Autodesk Inventor part; units mm, degrees
(part 3 of 6)
  line L1057 (-22.5678, -22.0282) -> (-22.8077, -22.2961) construction
  spline S252 degree 2 poles (-22.8077, -22.2961) (-23.0757, -22.5921) (-23.5275, -22.5921) knots 0 0 0 1 1 1
  line L1058 (-22.8077, -22.2961) -> (-23.0757, -22.5921) construction
  line L1059 (-23.0757, -22.5921) -> (-23.5275, -22.5921) construction
  line L1060 (-23.5275, -22.5921) -> (-23.7675, -22.5921)
  spline S253 degree 2 poles (-23.7675, -22.5921) (-24.2553, -22.5921) (-24.6272, -22.3041) knots 0 0 0 1 1 1
  line L1061 (-23.7675, -22.5921) -> (-24.2553, -22.5921) construction
  line L1062 (-24.2553, -22.5921) -> (-24.6272, -22.3041) construction
  spline S254 degree 2 poles (-24.6272, -22.3041) (-24.7272, -22.2282) (-24.7272, -22.1162) knots 0 0 0 1 1 1
  line L1063 (-24.6272, -22.3041) -> (-24.7272, -22.2282) construction
  line L1064 (-24.7272, -22.2282) -> (-24.7272, -22.1162) construction
  spline S255 degree 2 poles (-24.7272, -22.1162) (-24.7272, -22.0162) (-24.5832, -21.8683) (-24.4873, -21.8683) knots 0 0 0 1 2 2 2
  line L1065 (-24.7272, -22.1162) -> (-24.7272, -22.0162) construction
  line L1066 (-24.7272, -22.0162) -> (-24.5832, -21.8683) construction
  line L1067 (-24.5832, -21.8683) -> (-24.4873, -21.8683) construction
  spline S256 degree 2 poles (-24.4873, -21.8683) (-24.4113, -21.8683) (-24.3393, -21.9202) knots 0 0 0 1 1 1
  line L1068 (-24.4873, -21.8683) -> (-24.4113, -21.8683) construction
  line L1069 (-24.4113, -21.8683) -> (-24.3393, -21.9202) construction
  spline S257 degree 2 poles (-24.3393, -21.9202) (-24.0914, -22.1122) (-23.7675, -22.1122) knots 0 0 0 1 1 1
  line L1070 (-24.3393, -21.9202) -> (-24.0914, -22.1122) construction
  line L1071 (-24.0914, -22.1122) -> (-23.7675, -22.1122) construction
  line L1072 (-23.7675, -22.1122) -> (-23.5275, -22.1122)
  spline S258 degree 2 poles (-23.5275, -22.1122) (-23.2996, -22.1122) (-23.1676, -21.9602) knots 0 0 0 1 1 1
  line L1073 (-23.5275, -22.1122) -> (-23.2996, -22.1122) construction
  line L1074 (-23.2996, -22.1122) -> (-23.1676, -21.9602) construction
  spline S259 degree 2 poles (-23.1676, -21.9602) (-23.0477, -21.8243) (-23.0477, -21.6283) knots 0 0 0 1 1 1
  line L1075 (-23.1676, -21.9602) -> (-23.0477, -21.8243) construction
  line L1076 (-23.0477, -21.8243) -> (-23.0477, -21.6283) construction
  spline S260 degree 2 poles (-23.0477, -21.6283) (-23.0477, -21.2005) (-23.4635, -21.1565) knots 0 0 0 1 1 1
  line L1077 (-23.0477, -21.6283) -> (-23.0477, -21.2005) construction
  line L1078 (-23.0477, -21.2005) -> (-23.4635, -21.1565) construction
  line L1079 (-23.4635, -21.1565) -> (-23.7635, -21.1565)
  spline S261 degree 2 poles (10.7013, -8.7285) (10.4614, -8.7285) (10.4614, -8.4886) knots 0 0 0 1 1 1
  line L1080 (10.7013, -8.7285) -> (10.4614, -8.7285) construction
  line L1081 (10.4614, -8.7285) -> (10.4614, -8.4886) construction
  line L1082 (10.4614, -8.4886) -> (10.4614, -6.3372)
  spline S262 degree 2 poles (10.4614, -6.3372) (10.4614, -6.1413) (10.1815, -5.8573) (9.9855, -5.8573) knots 0 0 0 1 2 2 2
  line L1083 (10.4614, -6.3372) -> (10.4614, -6.1413) construction
  line L1084 (10.4614, -6.1413) -> (10.1815, -5.8573) construction
  line L1085 (10.1815, -5.8573) -> (9.9855, -5.8573) construction
  spline S263 degree 2 poles (9.0298, -8.4886) (9.0298, -8.7285) (8.7899, -8.7285) knots 0 0 0 1 1 1
  line L1086 (9.0298, -8.4886) -> (9.0298, -8.7285) construction
  line L1087 (9.0298, -8.7285) -> (8.7899, -8.7285) construction
  spline S264 degree 2 poles (8.7899, -8.7285) (8.5499, -8.7285) (8.5499, -8.4886) knots 0 0 0 1 1 1
  line L1088 (8.7899, -8.7285) -> (8.5499, -8.7285) construction
  line L1089 (8.5499, -8.7285) -> (8.5499, -8.4886) construction
  line L1090 (8.5499, -8.4886) -> (8.5499, -5.6174)
  spline S265 degree 2 poles (8.5499, -5.6174) (8.5499, -5.3775) (8.7899, -5.3775) knots 0 0 0 1 1 1
  line L1091 (8.5499, -5.6174) -> (8.5499, -5.3775) construction
  line L1092 (8.5499, -5.3775) -> (8.7899, -5.3775) construction
  line L1093 (8.7899, -5.3775) -> (9.9855, -5.3775)
  spline S266 degree 2 poles (9.9855, -5.3775) (10.3814, -5.3775) (10.9413, -5.9373) (10.9413, -6.3332) knots 0 0 0 1 2 2 2
  line L1094 (9.9855, -5.3775) -> (10.3814, -5.3775) construction
  line L1095 (10.3814, -5.3775) -> (10.9413, -5.9373) construction
  line L1096 (10.9413, -5.9373) -> (10.9413, -6.3332) construction
  line L1097 (10.9413, -6.3332) -> (10.9413, -8.4886)
  spline S267 degree 2 poles (10.9413, -8.4886) (10.9413, -8.7285) (10.7013, -8.7285) knots 0 0 0 1 1 1
  line L1098 (10.9413, -8.4886) -> (10.9413, -8.7285) construction
  line L1099 (10.9413, -8.7285) -> (10.7013, -8.7285) construction
  spline S268 degree 2 poles (6.6345, -8.2487) (6.8304, -8.2487) (7.1103, -7.9647) (7.1103, -7.7688) knots 0 0 0 1 2 2 2
  line L1100 (6.6345, -8.2487) -> (6.8304, -8.2487) construction
  line L1101 (6.8304, -8.2487) -> (7.1103, -7.9647) construction
  line L1102 (7.1103, -7.9647) -> (7.1103, -7.7688) construction
  spline S269 degree 2 poles (6.1546, -5.8573) (5.9587, -5.8573) (5.6787, -6.1413) (5.6787, -6.3372) knots 0 0 0 1 2 2 2
  line L1103 (6.1546, -5.8573) -> (5.9587, -5.8573) construction
  line L1104 (5.9587, -5.8573) -> (5.6787, -6.1413) construction
  line L1105 (5.6787, -6.1413) -> (5.6787, -6.3372) construction
  line L1106 (5.6787, -6.3372) -> (5.6787, -7.7688)
  spline S270 degree 2 poles (5.6787, -7.7688) (5.6787, -7.9647) (5.9587, -8.2487) (6.1546, -8.2487) knots 0 0 0 1 2 2 2
  line L1107 (5.6787, -7.7688) -> (5.6787, -7.9647) construction
  line L1108 (5.6787, -7.9647) -> (5.9587, -8.2487) construction
  line L1109 (5.9587, -8.2487) -> (6.1546, -8.2487) construction
  line L1110 (6.1546, -8.2487) -> (6.6345, -8.2487)
  line L1111 (6.6345, -8.7285) -> (6.1546, -8.7285)
  spline S271 degree 2 poles (6.1546, -8.7285) (5.7627, -8.7285) (5.1989, -8.1687) (5.1989, -7.7728) knots 0 0 0 1 2 2 2
  line L1112 (6.1546, -8.7285) -> (5.7627, -8.7285) construction
  line L1113 (5.7627, -8.7285) -> (5.1989, -8.1687) construction
  line L1114 (5.1989, -8.1687) -> (5.1989, -7.7728) construction
  line L1115 (5.1989, -7.7728) -> (5.1989, -6.3332)
  spline S272 degree 2 poles (5.1989, -6.3332) (5.1989, -5.9373) (5.7627, -5.3775) (6.1546, -5.3775) knots 0 0 0 1 2 2 2
  line L1116 (5.1989, -6.3332) -> (5.1989, -5.9373) construction
  line L1117 (5.1989, -5.9373) -> (5.7627, -5.3775) construction
  line L1118 (5.7627, -5.3775) -> (6.1546, -5.3775) construction
  line L1119 (6.1546, -5.3775) -> (7.3503, -5.3775)
  spline S273 degree 2 poles (7.3503, -5.3775) (7.5902, -5.3775) (7.5902, -5.6174) knots 0 0 0 1 1 1
  line L1120 (7.3503, -5.3775) -> (7.5902, -5.3775) construction
  line L1121 (7.5902, -5.3775) -> (7.5902, -5.6174) construction
  line L1122 (7.5902, -5.6174) -> (7.5902, -7.7648)
  spline S274 degree 2 poles (7.5902, -7.7648) (7.5902, -8.1247) (7.9261, -8.2687) knots 0 0 0 1 1 1
  line L1123 (7.5902, -7.7648) -> (7.5902, -8.1247) construction
  line L1124 (7.5902, -8.1247) -> (7.9261, -8.2687) construction
  spline S275 degree 2 poles (7.9261, -8.2687) (8.0741, -8.3286) (8.0741, -8.4806) knots 0 0 0 1 1 1
  line L1125 (7.9261, -8.2687) -> (8.0741, -8.3286) construction
  line L1126 (8.0741, -8.3286) -> (8.0741, -8.4806) construction
  spline S276 degree 2 poles (8.0741, -8.4806) (8.0741, -8.5806) (7.9381, -8.7325) (7.8381, -8.7325) knots 0 0 0 1 2 2 2
  line L1127 (8.0741, -8.4806) -> (8.0741, -8.5806) construction
  line L1128 (8.0741, -8.5806) -> (7.9381, -8.7325) construction
  line L1129 (7.9381, -8.7325) -> (7.8381, -8.7325) construction
  spline S277 degree 2 poles (7.8381, -8.7325) (7.7861, -8.7325) (7.7342, -8.7085) knots 0 0 0 1 1 1
  line L1130 (7.8381, -8.7325) -> (7.7861, -8.7325) construction
  line L1131 (7.7861, -8.7325) -> (7.7342, -8.7085) construction
  spline S278 degree 2 poles (7.7342, -8.7085) (7.4942, -8.6046) (7.3463, -8.4126) knots 0 0 0 1 1 1
  line L1132 (7.7342, -8.7085) -> (7.4942, -8.6046) construction
  line L1133 (7.4942, -8.6046) -> (7.3463, -8.4126) construction
  spline S279 degree 2 poles (7.3463, -8.4126) (7.0583, -8.7285) (6.6345, -8.7285) knots 0 0 0 1 1 1
  line L1134 (7.3463, -8.4126) -> (7.0583, -8.7285) construction
  line L1135 (7.0583, -8.7285) -> (6.6345, -8.7285) construction
  spline S280 degree 2 poles (8.5987, 1.0626) (8.3588, 1.0626) (8.3588, 1.3026) knots 0 0 0 1 1 1
  line L1136 (8.5987, 1.0626) -> (8.3588, 1.0626) construction
  line L1137 (8.3588, 1.0626) -> (8.3588, 1.3026) construction
  line L1138 (8.3588, 1.3026) -> (8.3588, 3.454)
  spline S281 degree 2 poles (8.3588, 3.454) (8.3588, 3.6499) (8.0788, 3.9338) (7.8829, 3.9338) knots 0 0 0 1 2 2 2
  line L1139 (8.3588, 3.454) -> (8.3588, 3.6499) construction
  line L1140 (8.3588, 3.6499) -> (8.0788, 3.9338) construction
  line L1141 (8.0788, 3.9338) -> (7.8829, 3.9338) construction
  spline S282 degree 2 poles (6.9272, 1.3026) (6.9272, 1.0626) (6.6872, 1.0626) knots 0 0 0 1 1 1
  line L1142 (6.9272, 1.3026) -> (6.9272, 1.0626) construction
  line L1143 (6.9272, 1.0626) -> (6.6872, 1.0626) construction
  spline S283 degree 2 poles (6.6872, 1.0626) (6.4473, 1.0626) (6.4473, 1.3026) knots 0 0 0 1 1 1
  line L1144 (6.6872, 1.0626) -> (6.4473, 1.0626) construction
  line L1145 (6.4473, 1.0626) -> (6.4473, 1.3026) construction
  line L1146 (6.4473, 1.3026) -> (6.4473, 4.1738)
  spline S284 degree 2 poles (6.4473, 4.1738) (6.4473, 4.4137) (6.6872, 4.4137) knots 0 0 0 1 1 1
  line L1147 (6.4473, 4.1738) -> (6.4473, 4.4137) construction
  line L1148 (6.4473, 4.4137) -> (6.6872, 4.4137) construction
  line L1149 (6.6872, 4.4137) -> (7.8829, 4.4137)
  spline S285 degree 2 poles (7.8829, 4.4137) (8.2788, 4.4137) (8.8386, 3.8539) (8.8386, 3.458) knots 0 0 0 1 2 2 2
  line L1150 (7.8829, 4.4137) -> (8.2788, 4.4137) construction
  line L1151 (8.2788, 4.4137) -> (8.8386, 3.8539) construction
  line L1152 (8.8386, 3.8539) -> (8.8386, 3.458) construction
  line L1153 (8.8386, 3.458) -> (8.8386, 1.3026)
  spline S286 degree 2 poles (8.8386, 1.3026) (8.8386, 1.0626) (8.5987, 1.0626) knots 0 0 0 1 1 1
  line L1154 (8.8386, 1.3026) -> (8.8386, 1.0626) construction
  line L1155 (8.8386, 1.0626) -> (8.5987, 1.0626) construction
  spline S287 degree 2 poles (-14.2805, -7.629) (-14.6764, -7.629) (-15.2362, -7.0692) (-15.2362, -6.6733) knots 0 0 0 1 2 2 2
  line L1156 (-14.2805, -7.629) -> (-14.6764, -7.629) construction
  line L1157 (-14.6764, -7.629) -> (-15.2362, -7.0692) construction
  line L1158 (-15.2362, -7.0692) -> (-15.2362, -6.6733) construction
  line L1159 (-15.2362, -6.6733) -> (-15.2362, -4.9978)
  spline S288 degree 2 poles (-15.2362, -4.9978) (-15.2362, -4.7578) (-14.9963, -4.7578) knots 0 0 0 1 1 1
  line L1160 (-15.2362, -4.9978) -> (-15.2362, -4.7578) construction
  line L1161 (-15.2362, -4.7578) -> (-14.9963, -4.7578) construction
  spline S289 degree 2 poles (-14.9963, -4.7578) (-14.7563, -4.7578) (-14.7563, -4.9978) knots 0 0 0 1 1 1
  line L1162 (-14.9963, -4.7578) -> (-14.7563, -4.7578) construction
  line L1163 (-14.7563, -4.7578) -> (-14.7563, -4.9978) construction
  line L1164 (-14.7563, -4.9978) -> (-14.7563, -6.6693)
  spline S290 degree 2 poles (-14.7563, -6.6693) (-14.7563, -6.8652) (-14.4724, -7.1491) (-14.2765, -7.1491) knots 0 0 0 1 2 2 2
  line L1165 (-14.7563, -6.6693) -> (-14.7563, -6.8652) construction
  line L1166 (-14.7563, -6.8652) -> (-14.4724, -7.1491) construction
  line L1167 (-14.4724, -7.1491) -> (-14.2765, -7.1491) construction
  spline S291 degree 2 poles (-12.8449, -4.9978) (-12.8449, -4.7578) (-12.6049, -4.7578) knots 0 0 0 1 1 1
  line L1168 (-12.8449, -4.9978) -> (-12.8449, -4.7578) construction
  line L1169 (-12.8449, -4.7578) -> (-12.6049, -4.7578) construction
  spline S292 degree 2 poles (-12.6049, -4.7578) (-12.365, -4.7578) (-12.365, -4.9978) knots 0 0 0 1 1 1
  line L1170 (-12.6049, -4.7578) -> (-12.365, -4.7578) construction
  line L1171 (-12.365, -4.7578) -> (-12.365, -4.9978) construction
  line L1172 (-12.365, -4.9978) -> (-12.365, -8.5887)
  spline S293 degree 2 poles (-12.365, -8.5887) (-12.365, -8.9846) (-12.9249, -9.5445) (-13.3207, -9.5445) knots 0 0 0 1 2 2 2
  line L1173 (-12.365, -8.5887) -> (-12.365, -8.9846) construction
  line L1174 (-12.365, -8.9846) -> (-12.9249, -9.5445) construction
  line L1175 (-12.9249, -9.5445) -> (-13.3207, -9.5445) construction
  line L1176 (-13.3207, -9.5445) -> (-14.5164, -9.5445)
  spline S294 degree 2 poles (-14.5164, -9.5445) (-14.7563, -9.5445) (-14.7563, -9.3045) knots 0 0 0 1 1 1
  line L1177 (-14.5164, -9.5445) -> (-14.7563, -9.5445) construction
  line L1178 (-14.7563, -9.5445) -> (-14.7563, -9.3045) construction
  spline S295 degree 2 poles (-14.7563, -9.3045) (-14.7563, -9.0646) (-14.5164, -9.0646) knots 0 0 0 1 1 1
  line L1179 (-14.7563, -9.3045) -> (-14.7563, -9.0646) construction
  line L1180 (-14.7563, -9.0646) -> (-14.5164, -9.0646) construction
  line L1181 (-14.5164, -9.0646) -> (-13.3207, -9.0646)
  spline S296 degree 2 poles (-13.3207, -9.0646) (-13.1248, -9.0646) (-12.8449, -8.7807) (-12.8449, -8.5847) knots 0 0 0 1 2 2 2
  line L1182 (-13.3207, -9.0646) -> (-13.1248, -9.0646) construction
  line L1183 (-13.1248, -9.0646) -> (-12.8449, -8.7807) construction
  line L1184 (-12.8449, -8.7807) -> (-12.8449, -8.5847) construction
  spline S297 degree 2 poles (-20.2548, -6.6733) (-20.0189, -6.6733) (-20.0189, -6.9132) knots 0 0 0 1 1 1
  line L1185 (-20.2548, -6.6733) -> (-20.0189, -6.6733) construction
  line L1186 (-20.0189, -6.6733) -> (-20.0189, -6.9132) construction
  spline S298 degree 2 poles (-20.0189, -6.9132) (-20.0189, -7.1531) (-20.2548, -7.1531) knots 0 0 0 1 1 1
  line L1187 (-20.0189, -6.9132) -> (-20.0189, -7.1531) construction
  line L1188 (-20.0189, -7.1531) -> (-20.2548, -7.1531) construction
  spline S299 degree 2 poles (-19.7789, -9.0646) (-19.539, -9.0646) (-19.539, -9.3045) knots 0 0 0 1 1 1
  line L1189 (-19.7789, -9.0646) -> (-19.539, -9.0646) construction
  line L1190 (-19.539, -9.0646) -> (-19.539, -9.3045) construction
  spline S300 degree 2 poles (-19.539, -9.3045) (-19.539, -9.5445) (-19.7789, -9.5445) knots 0 0 0 1 1 1
  line L1191 (-19.539, -9.3045) -> (-19.539, -9.5445) construction
  line L1192 (-19.539, -9.5445) -> (-19.7789, -9.5445) construction
  line L1193 (-19.7789, -9.5445) -> (-21.6984, -9.5445)
  spline S301 degree 2 poles (-21.6984, -9.5445) (-21.9383, -9.5445) (-21.9383, -9.3205) knots 0 0 0 1 1 1
  line L1194 (-21.6984, -9.5445) -> (-21.9383, -9.5445) construction
  line L1195 (-21.9383, -9.5445) -> (-21.9383, -9.3205) construction
  line L1196 (-21.9383, -9.3205) -> (-21.9383, -4.9978)
  spline S302 degree 2 poles (-21.9383, -4.9978) (-21.9383, -4.7578) (-21.6984, -4.7578) knots 0 0 0 1 1 1
  line L1197 (-21.9383, -4.9978) -> (-21.9383, -4.7578) construction
  line L1198 (-21.9383, -4.7578) -> (-21.6984, -4.7578) construction
  line L1199 (-21.6984, -4.7578) -> (-19.7789, -4.7578)
  spline S303 degree 2 poles (-19.7789, -4.7578) (-19.539, -4.7578) (-19.539, -4.9978) knots 0 0 0 1 1 1
  line L1200 (-19.7789, -4.7578) -> (-19.539, -4.7578) construction
  line L1201 (-19.539, -4.7578) -> (-19.539, -4.9978) construction
  spline S304 degree 2 poles (-19.539, -4.9978) (-19.539, -5.2377) (-19.7789, -5.2377) knots 0 0 0 1 1 1
  line L1202 (-19.539, -4.9978) -> (-19.539, -5.2377) construction
  line L1203 (-19.539, -5.2377) -> (-19.7789, -5.2377) construction
  spline S305 degree 2 poles (-19.9181, 7.2042) (-20.418, 7.2042) (-21.1178, 7.904) (-21.1178, 8.3999) knots 0 0 0 1 2 2 2
  line L1204 (-19.9181, 7.2042) -> (-20.418, 7.2042) construction
  line L1205 (-20.418, 7.2042) -> (-21.1178, 7.904) construction
  line L1206 (-21.1178, 7.904) -> (-21.1178, 8.3999) construction
  line L1207 (-21.1178, 8.3999) -> (-21.1178, 10.7952)
  spline S306 degree 2 poles (-21.1178, 10.7952) (-21.1178, 11.287) (-20.418, 11.9909) (-19.9181, 11.9909) knots 0 0 0 1 2 2 2
  line L1208 (-21.1178, 10.7952) -> (-21.1178, 11.287) construction
  line L1209 (-21.1178, 11.287) -> (-20.418, 11.9909) construction
  line L1210 (-20.418, 11.9909) -> (-19.9181, 11.9909) construction
  line L1211 (-19.9181, 11.9909) -> (-18.9624, 11.9909)
  spline S307 degree 2 poles (-18.9624, 11.9909) (-18.7225, 11.9909) (-18.7225, 11.7509) knots 0 0 0 1 1 1
  line L1212 (-18.9624, 11.9909) -> (-18.7225, 11.9909) construction
  line L1213 (-18.7225, 11.9909) -> (-18.7225, 11.7509) construction
  spline S308 degree 2 poles (-18.7225, 11.7509) (-18.7225, 11.511) (-18.9624, 11.511) knots 0 0 0 1 1 1
  line L1214 (-18.7225, 11.7509) -> (-18.7225, 11.511) construction
  line L1215 (-18.7225, 11.511) -> (-18.9624, 11.511) construction
  line L1216 (-18.9624, 11.511) -> (-19.9181, 11.511)
  spline S309 degree 2 poles (-19.9181, 11.511) (-20.218, 11.511) (-20.6379, 11.0911) (-20.6379, 10.7952) knots 0 0 0 1 2 2 2
  line L1217 (-19.9181, 11.511) -> (-20.218, 11.511) construction
  line L1218 (-20.218, 11.511) -> (-20.6379, 11.0911) construction
  line L1219 (-20.6379, 11.0911) -> (-20.6379, 10.7952) construction
  line L1220 (-20.6379, 10.7952) -> (-20.6379, 8.3999)
  spline S310 degree 2 poles (-20.6379, 8.3999) (-20.6379, 8.1039) (-20.218, 7.6841) (-19.9181, 7.6841) knots 0 0 0 1 2 2 2
  line L1221 (-20.6379, 8.3999) -> (-20.6379, 8.1039) construction
  line L1222 (-20.6379, 8.1039) -> (-20.218, 7.6841) construction
  line L1223 (-20.218, 7.6841) -> (-19.9181, 7.6841) construction
  line L1224 (-19.9181, 7.6841) -> (-18.9624, 7.6841)
  spline S311 degree 2 poles (-18.9624, 7.6841) (-18.7225, 7.6841) (-18.7225, 7.4441) knots 0 0 0 1 1 1
  line L1225 (-18.9624, 7.6841) -> (-18.7225, 7.6841) construction
  line L1226 (-18.7225, 7.6841) -> (-18.7225, 7.4441) construction
  spline S312 degree 2 poles (-18.7225, 7.4441) (-18.7225, 7.2042) (-18.9624, 7.2042) knots 0 0 0 1 1 1
  line L1227 (-18.7225, 7.4441) -> (-18.7225, 7.2042) construction
  line L1228 (-18.7225, 7.2042) -> (-18.9624, 7.2042) construction
  line L1229 (-18.9624, 7.2042) -> (-19.9181, 7.2042)
  spline S313 degree 2 poles (-10.2251, 1.4084) (-10.0292, 1.4084) (-9.7493, 1.6923) (-9.7493, 1.8882) knots 0 0 0 1 2 2 2
  line L1230 (-10.2251, 1.4084) -> (-10.0292, 1.4084) construction
  line L1231 (-10.0292, 1.4084) -> (-9.7493, 1.6923) construction
  line L1232 (-9.7493, 1.6923) -> (-9.7493, 1.8882) construction
  line L1233 (-9.7493, 1.8882) -> (-9.7493, 3.3198)
  spline S314 degree 2 poles (-9.7493, 3.3198) (-9.7493, 3.5158) (-10.0292, 3.7997) (-10.2251, 3.7997) knots 0 0 0 1 2 2 2
  line L1234 (-9.7493, 3.3198) -> (-9.7493, 3.5158) construction
  line L1235 (-9.7493, 3.5158) -> (-10.0292, 3.7997) construction
  line L1236 (-10.0292, 3.7997) -> (-10.2251, 3.7997) construction
  spline S315 degree 2 poles (-11.1809, -0.2671) (-11.1809, -0.5071) (-11.4208, -0.5071) knots 0 0 0 1 1 1
  line L1237 (-11.1809, -0.2671) -> (-11.1809, -0.5071) construction
  line L1238 (-11.1809, -0.5071) -> (-11.4208, -0.5071) construction
  spline S316 degree 2 poles (-11.4208, -0.5071) (-11.6607, -0.5071) (-11.6607, -0.2671) knots 0 0 0 1 1 1
  line L1239 (-11.4208, -0.5071) -> (-11.6607, -0.5071) construction
  line L1240 (-11.6607, -0.5071) -> (-11.6607, -0.2671) construction
  line L1241 (-11.6607, -0.2671) -> (-11.6607, 4.0396)
  spline S317 degree 2 poles (-11.6607, 4.0396) (-11.6607, 4.2796) (-11.4208, 4.2796) knots 0 0 0 1 1 1
  line L1242 (-11.6607, 4.0396) -> (-11.6607, 4.2796) construction
  line L1243 (-11.6607, 4.2796) -> (-11.4208, 4.2796) construction
  line L1244 (-11.4208, 4.2796) -> (-10.2251, 4.2796)
  spline S318 degree 2 poles (-10.2251, 4.2796) (-9.8293, 4.2796) (-9.2694, 3.7197) (-9.2694, 3.3238) knots 0 0 0 1 2 2 2
  line L1245 (-10.2251, 4.2796) -> (-9.8293, 4.2796) construction
  line L1246 (-9.8293, 4.2796) -> (-9.2694, 3.7197) construction
  line L1247 (-9.2694, 3.7197) -> (-9.2694, 3.3238) construction
  line L1248 (-9.2694, 3.3238) -> (-9.2694, 1.8842)
  spline S319 degree 2 poles (-9.2694, 1.8842) (-9.2694, 1.4884) (-9.8293, 0.9285) (-10.2251, 0.9285) knots 0 0 0 1 2 2 2
  line L1249 (-9.2694, 1.8842) -> (-9.2694, 1.4884) construction
  line L1250 (-9.2694, 1.4884) -> (-9.8293, 0.9285) construction
  line L1251 (-9.8293, 0.9285) -> (-10.2251, 0.9285) construction
  spline S320 degree 2 poles (-19.8024, 4.0396) (-19.8024, 4.2796) (-19.5625, 4.2796) knots 0 0 0 1 1 1
  line L1252 (-19.8024, 4.0396) -> (-19.8024, 4.2796) construction
  line L1253 (-19.8024, 4.2796) -> (-19.5625, 4.2796) construction
  spline S321 degree 2 poles (-19.5625, 4.2796) (-19.3226, 4.2796) (-19.3226, 4.0396) knots 0 0 0 1 1 1
  line L1254 (-19.5625, 4.2796) -> (-19.3226, 4.2796) construction
  line L1255 (-19.3226, 4.2796) -> (-19.3226, 4.0396) construction
  line L1256 (-19.3226, 4.0396) -> (-19.3226, 1.1685)
  spline S322 degree 2 poles (-19.3226, 1.1685) (-19.3226, 0.9285) (-19.5625, 0.9285) knots 0 0 0 1 1 1
  line L1257 (-19.3226, 1.1685) -> (-19.3226, 0.9285) construction
  line L1258 (-19.3226, 0.9285) -> (-19.5625, 0.9285) construction
  spline S323 degree 2 poles (-19.5625, 0.9285) (-19.8024, 0.9285) (-19.8024, 1.1685) knots 0 0 0 1 1 1
  line L1259 (-19.5625, 0.9285) -> (-19.8024, 0.9285) construction
  line L1260 (-19.8024, 0.9285) -> (-19.8024, 1.1685) construction
  spline S324 degree 2 poles (-21.234, 1.1685) (-21.234, 0.9285) (-21.474, 0.9285) knots 0 0 0 1 1 1
  line L1261 (-21.234, 1.1685) -> (-21.234, 0.9285) construction
  line L1262 (-21.234, 0.9285) -> (-21.474, 0.9285) construction
  spline S325 degree 2 poles (-21.474, 0.9285) (-21.7139, 0.9285) (-21.7139, 1.1685) knots 0 0 0 1 1 1
  line L1263 (-21.474, 0.9285) -> (-21.7139, 0.9285) construction
  line L1264 (-21.7139, 0.9285) -> (-21.7139, 1.1685) construction
  line L1265 (-21.7139, 1.1685) -> (-21.7139, 4.0396)
  spline S326 degree 2 poles (-21.7139, 4.0396) (-21.7139, 4.2796) (-21.474, 4.2796) knots 0 0 0 1 1 1
  line L1266 (-21.7139, 4.0396) -> (-21.7139, 4.2796) construction
  line L1267 (-21.7139, 4.2796) -> (-21.474, 4.2796) construction
  spline S327 degree 2 poles (-21.474, 4.2796) (-21.234, 4.2796) (-21.234, 4.0396) knots 0 0 0 1 1 1
  line L1268 (-21.474, 4.2796) -> (-21.234, 4.2796) construction
  line L1269 (-21.234, 4.2796) -> (-21.234, 4.0396) construction
  line L1270 (-18.0648, 28.7283) -> (-16.6292, 28.7283)
  spline S328 degree 2 poles (-16.6292, 28.7283) (-16.3893, 28.7283) (-16.3893, 28.4883) knots 0 0 0 1 1 1
  line L1271 (-16.6292, 28.7283) -> (-16.3893, 28.7283) construction
  line L1272 (-16.3893, 28.7283) -> (-16.3893, 28.4883) construction
  spline S329 degree 2 poles (-22.3312, 37.5726) (-22.4482, 37.5726) (-22.6239, 37.7483) (-22.6239, 37.8654) knots 0 0 0 1 2 2 2
  line L1273 (-22.3312, 37.5726) -> (-22.4482, 37.5726) construction
  line L1274 (-22.4482, 37.5726) -> (-22.6239, 37.7483) construction
  line L1275 (-22.6239, 37.7483) -> (-22.6239, 37.8654) construction
  line L1276 (-22.6239, 37.8654) -> (-22.6239, 43.1196)
  spline S330 degree 2 poles (-22.6239, 43.1196) (-22.6239, 43.2367) (-22.4482, 43.4124) (-22.3312, 43.4124) knots 0 0 0 1 2 2 2
  line L1277 (-22.6239, 43.1196) -> (-22.6239, 43.2367) construction
  line L1278 (-22.6239, 43.2367) -> (-22.4482, 43.4124) construction
  line L1279 (-22.4482, 43.4124) -> (-22.3312, 43.4124) construction
  spline S331 degree 2 poles (14.945, 104.9441) (14.9341, 104.5681) (14.9069, 103.8762) (14.8906, 103.5983) knots 0 0 0 1 2 2 2
  line L1280 (14.945, 104.9441) -> (14.9341, 104.5681) construction
  line L1281 (14.9341, 104.5681) -> (14.9069, 103.8762) construction
  line L1282 (14.9069, 103.8762) -> (14.8906, 103.5983) construction
  spline S332 degree 2 poles (14.8906, 103.5983) (14.8633, 102.8899) (14.7325, 101.931) (14.6345, 101.6422) knots 0 0 0 1 2 2 2
  line L1283 (14.8906, 103.5983) -> (14.8633, 102.8899) construction
  line L1284 (14.8633, 102.8899) -> (14.7325, 101.931) construction
  line L1285 (14.7325, 101.931) -> (14.6345, 101.6422) construction
  spline S333 degree 2 poles (14.6345, 101.6422) (14.5364, 101.3425) (14.2966, 101.0101) (14.1441, 100.8739) knots 0 0 0 1 2 2 2
  line L1286 (14.6345, 101.6422) -> (14.5364, 101.3425) construction
  line L1287 (14.5364, 101.3425) -> (14.2966, 101.0101) construction
  line L1288 (14.2966, 101.0101) -> (14.1441, 100.8739) construction
  spline S334 degree 2 poles (14.1441, 100.8739) (13.9915, 100.7377) (13.6428, 100.6015) (13.4194, 100.6015) knots 0 0 0 1 2 2 2
  line L1289 (14.1441, 100.8739) -> (13.9915, 100.7377) construction
  line L1290 (13.9915, 100.7377) -> (13.6428, 100.6015) construction
  line L1291 (13.6428, 100.6015) -> (13.4194, 100.6015) construction
  spline S335 degree 2 poles (13.4194, 100.6015) (13.3486, 100.6015) (13.1197, 100.6124) (13.0761, 100.6124) knots 0 0 0 1 2 2 2
  line L1292 (13.4194, 100.6015) -> (13.3486, 100.6015) construction
  line L1293 (13.3486, 100.6015) -> (13.1197, 100.6124) construction
  line L1294 (13.1197, 100.6124) -> (13.0761, 100.6124) construction
  spline S336 degree 2 poles (13.1197, 101.3534) (13.1524, 101.3534) (13.2233, 101.3425) (13.2668, 101.3425) knots 0 0 0 1 2 2 2
  line L1295 (13.1197, 101.3534) -> (13.1524, 101.3534) construction
  line L1296 (13.1524, 101.3534) -> (13.2233, 101.3425) construction
  line L1297 (13.2233, 101.3425) -> (13.2668, 101.3425) construction
  spline S337 degree 2 poles (13.2668, 101.3425) (13.3758, 101.3425) (13.5829, 101.4079) (13.6646, 101.4896) knots 0 0 0 1 2 2 2
  line L1298 (13.2668, 101.3425) -> (13.3758, 101.3425) construction
  line L1299 (13.3758, 101.3425) -> (13.5829, 101.4079) construction
  line L1300 (13.5829, 101.4079) -> (13.6646, 101.4896) construction
  spline S338 degree 2 poles (13.6646, 101.4896) (13.888, 101.713) (14.095, 102.8191) (14.1386, 103.8162) knots 0 0 0 1 2 2 2
  line L1301 (13.6646, 101.4896) -> (13.888, 101.713) construction
  line L1302 (13.888, 101.713) -> (14.095, 102.8191) construction
  line L1303 (14.095, 102.8191) -> (14.1386, 103.8162) construction
  spline S339 degree 2 poles (14.1386, 103.8162) (14.1604, 104.1867) (14.1931, 105.1947) (14.204, 105.6579) knots 0 0 0 1 2 2 2
  line L1304 (14.1386, 103.8162) -> (14.1604, 104.1867) construction
  line L1305 (14.1604, 104.1867) -> (14.1931, 105.1947) construction
  line L1306 (14.1931, 105.1947) -> (14.204, 105.6579) construction
  spline S340 degree 2 poles (10.5043, 101.2008) (11.1582, 101.2008) (11.8774, 102.1653) (11.8774, 103.1351) knots 0 0 0 1 2 2 2
  line L1307 (10.5043, 101.2008) -> (11.1582, 101.2008) construction
  line L1308 (11.1582, 101.2008) -> (11.8774, 102.1653) construction
  line L1309 (11.8774, 102.1653) -> (11.8774, 103.1351) construction
  spline S341 degree 2 poles (11.8774, 103.1351) (11.8774, 104.1159) (11.1636, 105.0694) (10.5043, 105.0694) knots 0 0 0 1 2 2 2
  line L1310 (11.8774, 103.1351) -> (11.8774, 104.1159) construction
  line L1311 (11.8774, 104.1159) -> (11.1636, 105.0694) construction
  line L1312 (11.1636, 105.0694) -> (10.5043, 105.0694) construction
  spline S342 degree 2 poles (10.5043, 105.0694) (9.8451, 105.0694) (9.1258, 104.1159) (9.1258, 103.1351) knots 0 0 0 1 2 2 2
  line L1313 (10.5043, 105.0694) -> (9.8451, 105.0694) construction
  line L1314 (9.8451, 105.0694) -> (9.1258, 104.1159) construction
  line L1315 (9.1258, 104.1159) -> (9.1258, 103.1351) construction
  spline S343 degree 2 poles (9.1258, 103.1351) (9.1258, 102.1816) (9.8451, 101.2008) (10.5043, 101.2008) knots 0 0 0 1 2 2 2
  line L1316 (9.1258, 103.1351) -> (9.1258, 102.1816) construction
  line L1317 (9.1258, 102.1816) -> (9.8451, 101.2008) construction
  line L1318 (9.8451, 101.2008) -> (10.5043, 101.2008) construction
  spline S344 degree 2 poles (10.5043, 100.4707) (9.4527, 100.4707) (8.2486, 101.9037) (8.2486, 103.1351) knots 0 0 0 1 2 2 2
  line L1319 (10.5043, 100.4707) -> (9.4527, 100.4707) construction
  line L1320 (9.4527, 100.4707) -> (8.2486, 101.9037) construction
  line L1321 (8.2486, 101.9037) -> (8.2486, 103.1351) construction
  spline S345 degree 2 poles (8.2486, 103.1351) (8.2486, 104.3992) (9.4909, 105.7995) (10.5043, 105.7995) knots 0 0 0 1 2 2 2
  line L1322 (8.2486, 103.1351) -> (8.2486, 104.3992) construction
  line L1323 (8.2486, 104.3992) -> (9.4909, 105.7995) construction
  line L1324 (9.4909, 105.7995) -> (10.5043, 105.7995) construction
  spline S346 degree 2 poles (10.5043, 105.7995) (11.5287, 105.7995) (12.7547, 104.4047) (12.7547, 103.1351) knots 0 0 0 1 2 2 2
  line L1325 (10.5043, 105.7995) -> (11.5287, 105.7995) construction
  line L1326 (11.5287, 105.7995) -> (12.7547, 104.4047) construction
  line L1327 (12.7547, 104.4047) -> (12.7547, 103.1351) construction
  spline S347 degree 2 poles (12.7547, 103.1351) (12.7547, 101.8601) (11.5287, 100.4707) (10.5043, 100.4707) knots 0 0 0 1 2 2 2
  line L1328 (12.7547, 103.1351) -> (12.7547, 101.8601) construction
  line L1329 (12.7547, 101.8601) -> (11.5287, 100.4707) construction
  line L1330 (11.5287, 100.4707) -> (10.5043, 100.4707) construction
  spline S348 degree 2 poles (5.4588, 101.2771) (6.1181, 101.2771) (6.8483, 102.247) (6.8483, 103.1733) knots 0 0 0 1 2 2 2
  line L1331 (5.4588, 101.2771) -> (6.1181, 101.2771) construction
  line L1332 (6.1181, 101.2771) -> (6.8483, 102.247) construction
  line L1333 (6.8483, 102.247) -> (6.8483, 103.1733) construction
  spline S349 degree 2 poles (6.8483, 103.1733) (6.8483, 104.0396) (6.2979, 104.9931) (5.6822, 104.9931) knots 0 0 0 1 2 2 2
  line L1334 (6.8483, 103.1733) -> (6.8483, 104.0396) construction
  line L1335 (6.8483, 104.0396) -> (6.2979, 104.9931) construction
  line L1336 (6.2979, 104.9931) -> (5.6822, 104.9931) construction
  spline S350 degree 2 poles (5.6822, 104.9931) (5.3226, 104.9931) (4.647, 104.6717) (4.3473, 104.421) knots 0 0 0 1 2 2 2
  line L1337 (5.6822, 104.9931) -> (5.3226, 104.9931) construction
  line L1338 (5.3226, 104.9931) -> (4.647, 104.6717) construction
  line L1339 (4.647, 104.6717) -> (4.3473, 104.421) construction
  line L1340 (4.3473, 104.421) -> (4.3473, 101.555)
  spline S351 degree 2 poles (4.3473, 101.555) (4.6797, 101.397) (5.1537, 101.2771) (5.4588, 101.2771) knots 0 0 0 1 2 2 2
  line L1341 (4.3473, 101.555) -> (4.6797, 101.397) construction
  line L1342 (4.6797, 101.397) -> (5.1537, 101.2771) construction
  line L1343 (5.1537, 101.2771) -> (5.4588, 101.2771) construction
  spline S352 degree 2 poles (5.6005, 100.5143) (5.2246, 100.5143) (4.647, 100.6887) (4.3473, 100.8685) knots 0 0 0 1 2 2 2
  line L1344 (5.6005, 100.5143) -> (5.2246, 100.5143) construction
  line L1345 (5.2246, 100.5143) -> (4.647, 100.6887) construction
  line L1346 (4.647, 100.6887) -> (4.3473, 100.8685) construction
  spline S353 degree 2 poles (4.3473, 105.1294) (4.6633, 105.4181) (5.4371, 105.7995) (5.8893, 105.7995) knots 0 0 0 1 2 2 2
  line L1347 (4.3473, 105.1294) -> (4.6633, 105.4181) construction
  line L1348 (4.6633, 105.4181) -> (5.4371, 105.7995) construction
  line L1349 (5.4371, 105.7995) -> (5.8893, 105.7995) construction
  spline S354 degree 2 poles (5.8893, 105.7995) (6.7556, 105.7995) (7.7255, 104.4265) (7.7255, 103.2713) knots 0 0 0 1 2 2 2
  line L1350 (5.8893, 105.7995) -> (6.7556, 105.7995) construction
  line L1351 (6.7556, 105.7995) -> (7.7255, 104.4265) construction
  line L1352 (7.7255, 104.4265) -> (7.7255, 103.2713) construction
  spline S355 degree 2 poles (7.7255, 103.2713) (7.7255, 102.0072) (6.5213, 100.5143) (5.6005, 100.5143) knots 0 0 0 1 2 2 2
  line L1353 (7.7255, 103.2713) -> (7.7255, 102.0072) construction
  line L1354 (7.7255, 102.0072) -> (6.5213, 100.5143) construction
  line L1355 (6.5213, 100.5143) -> (5.6005, 100.5143) construction
  spline S356 degree 2 poles (-9.1437, 101.2008) (-8.4898, 101.2008) (-7.7706, 102.1653) (-7.7706, 103.1351) knots 0 0 0 1 2 2 2
  line L1356 (-9.1437, 101.2008) -> (-8.4898, 101.2008) construction
  line L1357 (-8.4898, 101.2008) -> (-7.7706, 102.1653) construction
  line L1358 (-7.7706, 102.1653) -> (-7.7706, 103.1351) construction
  spline S357 degree 2 poles (-7.7706, 103.1351) (-7.7706, 104.1159) (-8.4844, 105.0694) (-9.1437, 105.0694) knots 0 0 0 1 2 2 2
  line L1359 (-7.7706, 103.1351) -> (-7.7706, 104.1159) construction
  line L1360 (-7.7706, 104.1159) -> (-8.4844, 105.0694) construction
  line L1361 (-8.4844, 105.0694) -> (-9.1437, 105.0694) construction
  spline S358 degree 2 poles (-9.1437, 105.0694) (-9.803, 105.0694) (-10.5222, 104.1159) (-10.5222, 103.1351) knots 0 0 0 1 2 2 2
  line L1362 (-9.1437, 105.0694) -> (-9.803, 105.0694) construction
  line L1363 (-9.803, 105.0694) -> (-10.5222, 104.1159) construction
  line L1364 (-10.5222, 104.1159) -> (-10.5222, 103.1351) construction
  spline S359 degree 2 poles (-10.5222, 103.1351) (-10.5222, 102.1816) (-9.803, 101.2008) (-9.1437, 101.2008) knots 0 0 0 1 2 2 2
  line L1365 (-10.5222, 103.1351) -> (-10.5222, 102.1816) construction
  line L1366 (-10.5222, 102.1816) -> (-9.803, 101.2008) construction
  line L1367 (-9.803, 101.2008) -> (-9.1437, 101.2008) construction
  spline S360 degree 2 poles (-9.1437, 100.4707) (-10.1953, 100.4707) (-11.3995, 101.9037) (-11.3995, 103.1351) knots 0 0 0 1 2 2 2
  line L1368 (-9.1437, 100.4707) -> (-10.1953, 100.4707) construction
  line L1369 (-10.1953, 100.4707) -> (-11.3995, 101.9037) construction
  line L1370 (-11.3995, 101.9037) -> (-11.3995, 103.1351) construction
  spline S361 degree 2 poles (-11.3995, 103.1351) (-11.3995, 104.3992) (-10.1572, 105.7995) (-9.1437, 105.7995) knots 0 0 0 1 2 2 2
  line L1371 (-11.3995, 103.1351) -> (-11.3995, 104.3992) construction
  line L1372 (-11.3995, 104.3992) -> (-10.1572, 105.7995) construction
  line L1373 (-10.1572, 105.7995) -> (-9.1437, 105.7995) construction
  spline S362 degree 2 poles (-9.1437, 105.7995) (-8.1193, 105.7995) (-6.8934, 104.4047) (-6.8934, 103.1351) knots 0 0 0 1 2 2 2
  line L1374 (-9.1437, 105.7995) -> (-8.1193, 105.7995) construction
  line L1375 (-8.1193, 105.7995) -> (-6.8934, 104.4047) construction
  line L1376 (-6.8934, 104.4047) -> (-6.8934, 103.1351) construction
  spline S363 degree 2 poles (-6.8934, 103.1351) (-6.8934, 101.8601) (-8.1193, 100.4707) (-9.1437, 100.4707) knots 0 0 0 1 2 2 2
  line L1377 (-6.8934, 103.1351) -> (-6.8934, 101.8601) construction
  line L1378 (-6.8934, 101.8601) -> (-8.1193, 100.4707) construction
  line L1379 (-8.1193, 100.4707) -> (-9.1437, 100.4707) construction
  spline S364 degree 2 poles (-1.8953, 94.9906) (-1.6713, 94.9906) (-1.5394, 95.1385) knots 0 0 0 1 1 1
  line L1380 (-1.8953, 94.9906) -> (-1.6713, 94.9906) construction
  line L1381 (-1.6713, 94.9906) -> (-1.5394, 95.1385) construction
  spline S365 degree 2 poles (-1.5394, 95.1385) (-1.4194, 95.2745) (-1.4194, 95.4704) knots 0 0 0 1 1 1
  line L1382 (-1.5394, 95.1385) -> (-1.4194, 95.2745) construction
  line L1383 (-1.4194, 95.2745) -> (-1.4194, 95.4704) construction
  spline S366 degree 2 poles (-1.4194, 95.4704) (-1.4194, 95.6664) (-1.5394, 95.7983) knots 0 0 0 1 1 1
  line L1384 (-1.4194, 95.4704) -> (-1.4194, 95.6664) construction
  line L1385 (-1.4194, 95.6664) -> (-1.5394, 95.7983) construction
  spline S367 degree 2 poles (-1.5394, 95.7983) (-1.6713, 95.9463) (-1.8953, 95.9463) knots 0 0 0 1 1 1
  line L1386 (-1.5394, 95.7983) -> (-1.6713, 95.9463) construction
  line L1387 (-1.6713, 95.9463) -> (-1.8953, 95.9463) construction
  spline S368 degree 2 poles (-1.8953, 96.4262) (-1.4434, 96.4262) (-1.1795, 96.1263) knots 0 0 0 1 1 1
  line L1388 (-1.8953, 96.4262) -> (-1.4434, 96.4262) construction
  line L1389 (-1.4434, 96.4262) -> (-1.1795, 96.1263) construction
  spline S369 degree 2 poles (-1.1795, 96.1263) (-0.9395, 95.8583) (-0.9395, 95.4704) knots 0 0 0 1 1 1
  line L1390 (-1.1795, 96.1263) -> (-0.9395, 95.8583) construction
  line L1391 (-0.9395, 95.8583) -> (-0.9395, 95.4704) construction
  spline S370 degree 2 poles (-0.9395, 95.4704) (-0.9395, 95.0825) (-1.1795, 94.8066) knots 0 0 0 1 1 1
  line L1392 (-0.9395, 95.4704) -> (-0.9395, 95.0825) construction
  line L1393 (-0.9395, 95.0825) -> (-1.1795, 94.8066) construction
  spline S371 degree 2 poles (-1.1795, 94.8066) (-1.4434, 94.5107) (-1.8953, 94.5107) knots 0 0 0 1 1 1
  line L1394 (-1.1795, 94.8066) -> (-1.4434, 94.5107) construction
  line L1395 (-1.4434, 94.5107) -> (-1.8953, 94.5107) construction
  line L1396 (-1.8953, 94.5107) -> (-2.6151, 94.5107)
  spline S372 degree 2 poles (-2.6151, 94.5107) (-2.855, 94.5107) (-2.855, 94.7506) knots 0 0 0 1 1 1
  line L1397 (-2.6151, 94.5107) -> (-2.855, 94.5107) construction
  line L1398 (-2.855, 94.5107) -> (-2.855, 94.7506) construction
  line L1399 (-2.855, 94.7506) -> (-2.855, 97.6218)
  spline S373 degree 2 poles (-2.855, 97.6218) (-2.855, 97.8618) (-2.6151, 97.8618) knots 0 0 0 1 1 1
  line L1400 (-2.855, 97.6218) -> (-2.855, 97.8618) construction
  line L1401 (-2.855, 97.8618) -> (-2.6151, 97.8618) construction
  spline S374 degree 2 poles (-2.6151, 97.8618) (-2.3751, 97.8618) (-2.3751, 97.6218) knots 0 0 0 1 1 1
  line L1402 (-2.6151, 97.8618) -> (-2.3751, 97.8618) construction
  line L1403 (-2.3751, 97.8618) -> (-2.3751, 97.6218) construction
  spline S375 degree 2 poles (-13.8679, 94.7506) (-13.8679, 94.5107) (-14.1078, 94.5107) knots 0 0 0 1 1 1
  line L1404 (-13.8679, 94.7506) -> (-13.8679, 94.5107) construction
  line L1405 (-13.8679, 94.5107) -> (-14.1078, 94.5107) construction
  spline S376 degree 2 poles (-14.1078, 94.5107) (-14.3478, 94.5107) (-14.3478, 94.7506) knots 0 0 0 1 1 1
  line L1406 (-14.1078, 94.5107) -> (-14.3478, 94.5107) construction
  line L1407 (-14.3478, 94.5107) -> (-14.3478, 94.7506) construction
  line L1408 (-14.3478, 94.7506) -> (-14.3478, 97.6218)
  spline S377 degree 2 poles (-14.3478, 97.6218) (-14.3478, 97.8618) (-14.1078, 97.8618) knots 0 0 0 1 1 1
  line L1409 (-14.3478, 97.6218) -> (-14.3478, 97.8618) construction
  line L1410 (-14.3478, 97.8618) -> (-14.1078, 97.8618) construction
  line L1411 (-14.1078, 97.8618) -> (-11.9524, 97.8618)
  spline S378 degree 2 poles (-11.9524, 97.8618) (-11.5566, 97.8618) (-10.9967, 97.3019) (-10.9967, 96.906) knots 0 0 0 1 2 2 2
  line L1412 (-11.9524, 97.8618) -> (-11.5566, 97.8618) construction
  line L1413 (-11.5566, 97.8618) -> (-10.9967, 97.3019) construction
  line L1414 (-10.9967, 97.3019) -> (-10.9967, 96.906) construction
  line L1415 (-10.9967, 96.906) -> (-10.9967, 94.7506)
  spline S379 degree 2 poles (-10.9967, 94.7506) (-10.9967, 94.5107) (-11.2366, 94.5107) knots 0 0 0 1 1 1
  line L1416 (-10.9967, 94.7506) -> (-10.9967, 94.5107) construction
  line L1417 (-10.9967, 94.5107) -> (-11.2366, 94.5107) construction
  spline S380 degree 2 poles (-11.2366, 94.5107) (-11.4766, 94.5107) (-11.4766, 94.7506) knots 0 0 0 1 1 1
  line L1418 (-11.2366, 94.5107) -> (-11.4766, 94.5107) construction
  line L1419 (-11.4766, 94.5107) -> (-11.4766, 94.7506) construction
  line L1420 (-11.4766, 94.7506) -> (-11.4766, 96.902)
  spline S381 degree 2 poles (-11.4766, 96.902) (-11.4766, 97.098) (-11.7565, 97.3819) (-11.9524, 97.3819) knots 0 0 0 1 2 2 2
  line L1421 (-11.4766, 96.902) -> (-11.4766, 97.098) construction
  line L1422 (-11.4766, 97.098) -> (-11.7565, 97.3819) construction
  line L1423 (-11.7565, 97.3819) -> (-11.9524, 97.3819) construction
  spline S382 degree 2 poles (-12.4323, 94.7506) (-12.4323, 94.5107) (-12.6722, 94.5107) knots 0 0 0 1 1 1
  line L1424 (-12.4323, 94.7506) -> (-12.4323, 94.5107) construction
  line L1425 (-12.4323, 94.5107) -> (-12.6722, 94.5107) construction
  spline S383 degree 2 poles (-12.6722, 94.5107) (-12.9122, 94.5107) (-12.9122, 94.7506) knots 0 0 0 1 1 1
  line L1426 (-12.6722, 94.5107) -> (-12.9122, 94.5107) construction
  line L1427 (-12.9122, 94.5107) -> (-12.9122, 94.7506) construction
  line L1428 (-18.4186, 94.5107) -> (-19.6143, 94.5107)
  spline S384 degree 2 poles (-19.6143, 94.5107) (-20.0062, 94.5107) (-20.57, 95.0705) (-20.57, 95.4664) knots 0 0 0 1 2 2 2
  line L1429 (-19.6143, 94.5107) -> (-20.0062, 94.5107) construction
  line L1430 (-20.0062, 94.5107) -> (-20.57, 95.0705) construction
  line L1431 (-20.57, 95.0705) -> (-20.57, 95.4664) construction
  line L1432 (-20.57, 95.4664) -> (-20.57, 97.6218)
  spline S385 degree 2 poles (-20.57, 97.6218) (-20.57, 97.8618) (-20.3301, 97.8618) knots 0 0 0 1 1 1
  line L1433 (-20.57, 97.6218) -> (-20.57, 97.8618) construction
  line L1434 (-20.57, 97.8618) -> (-20.3301, 97.8618) construction
  spline S386 degree 2 poles (-20.3301, 97.8618) (-20.0901, 97.8618) (-20.0901, 97.6218) knots 0 0 0 1 1 1
  line L1435 (-20.3301, 97.8618) -> (-20.0901, 97.8618) construction
  line L1436 (-20.0901, 97.8618) -> (-20.0901, 97.6218) construction
  line L1437 (-20.0901, 97.6218) -> (-20.0901, 95.4704)
  spline S387 degree 2 poles (-20.0901, 95.4704) (-20.0901, 95.2745) (-19.8102, 94.9906) (-19.6143, 94.9906) knots 0 0 0 1 2 2 2
  line L1438 (-20.0901, 95.4704) -> (-20.0901, 95.2745) construction
  line L1439 (-20.0901, 95.2745) -> (-19.8102, 94.9906) construction
  line L1440 (-19.8102, 94.9906) -> (-19.6143, 94.9906) construction
  spline S388 degree 2 poles (-18.6586, 97.6218) (-18.6586, 97.8618) (-18.4186, 97.8618) knots 0 0 0 1 1 1
  line L1441 (-18.6586, 97.6218) -> (-18.6586, 97.8618) construction
  line L1442 (-18.6586, 97.8618) -> (-18.4186, 97.8618) construction
  spline S389 degree 2 poles (-18.4186, 97.8618) (-18.1787, 97.8618) (-18.1787, 97.6218) knots 0 0 0 1 1 1
  line L1443 (-18.4186, 97.8618) -> (-18.1787, 97.8618) construction
  line L1444 (-18.1787, 97.8618) -> (-18.1787, 97.6218) construction
  line L1445 (-18.1787, 97.6218) -> (-18.1787, 94.7506)
  spline S390 degree 2 poles (-18.1787, 94.7506) (-18.1787, 94.5107) (-18.4186, 94.5107) knots 0 0 0 1 1 1
  line L1446 (-18.1787, 94.7506) -> (-18.1787, 94.5107) construction
  line L1447 (-18.1787, 94.5107) -> (-18.4186, 94.5107) construction
  circle A64 centre (0.0667, -82.7708) radius 10.9188
  circle A65 centre (0.0667, -82.7708) radius 11.8793
  spline S391 degree 2 poles (-22.4815, 94.5107) (-22.8734, 94.5107) (-23.4412, 95.0705) (-23.4412, 95.4664) knots 0 0 0 1 2 2 2
  line L1448 (-22.4815, 94.5107) -> (-22.8734, 94.5107) construction
  line L1449 (-22.8734, 94.5107) -> (-23.4412, 95.0705) construction
  line L1450 (-23.4412, 95.0705) -> (-23.4412, 95.4664) construction
  line L1451 (-23.4412, 95.4664) -> (-23.4412, 96.906)
  spline S392 degree 2 poles (-23.4412, 96.906) (-23.4412, 97.3019) (-22.8734, 97.8618) (-22.4815, 97.8618) knots 0 0 0 1 2 2 2
  line L1452 (-23.4412, 96.906) -> (-23.4412, 97.3019) construction
  line L1453 (-23.4412, 97.3019) -> (-22.8734, 97.8618) construction
  line L1454 (-22.8734, 97.8618) -> (-22.4815, 97.8618) construction
  line L1455 (-22.4815, 97.8618) -> (-21.7657, 97.8618)
  spline S393 degree 2 poles (-21.7657, 97.8618) (-21.5257, 97.8618) (-21.5257, 97.6218) knots 0 0 0 1 1 1
  line L1456 (-21.7657, 97.8618) -> (-21.5257, 97.8618) construction
  line L1457 (-21.5257, 97.8618) -> (-21.5257, 97.6218) construction
  spline S394 degree 2 poles (-21.5257, 97.6218) (-21.5257, 97.3819) (-21.7657, 97.3819) knots 0 0 0 1 1 1
  line L1458 (-21.5257, 97.6218) -> (-21.5257, 97.3819) construction
  line L1459 (-21.5257, 97.3819) -> (-21.7657, 97.3819) construction
  line L1460 (-21.7657, 97.3819) -> (-22.4815, 97.3819)
  spline S395 degree 2 poles (-22.4815, 97.3819) (-22.6774, 97.3819) (-22.9613, 97.098) (-22.9613, 96.902) knots 0 0 0 1 2 2 2
  line L1461 (-22.4815, 97.3819) -> (-22.6774, 97.3819) construction
  line L1462 (-22.6774, 97.3819) -> (-22.9613, 97.098) construction
  line L1463 (-22.9613, 97.098) -> (-22.9613, 96.902) construction
  line L1464 (-22.9613, 96.902) -> (-22.9613, 95.4704)
  spline S396 degree 2 poles (-22.9613, 95.4704) (-22.9613, 95.2745) (-22.6774, 94.9906) (-22.4815, 94.9906) knots 0 0 0 1 2 2 2
  line L1465 (-22.9613, 95.4704) -> (-22.9613, 95.2745) construction
  line L1466 (-22.9613, 95.2745) -> (-22.6774, 94.9906) construction
  line L1467 (-22.6774, 94.9906) -> (-22.4815, 94.9906) construction
  line L1468 (-22.4815, 94.9906) -> (-21.7657, 94.9906)
  spline S397 degree 2 poles (-21.7657, 94.9906) (-21.5257, 94.9906) (-21.5257, 94.7506) knots 0 0 0 1 1 1
  line L1469 (-21.7657, 94.9906) -> (-21.5257, 94.9906) construction
  line L1470 (-21.5257, 94.9906) -> (-21.5257, 94.7506) construction
  spline S398 degree 2 poles (-21.5257, 94.7506) (-21.5257, 94.5107) (-21.7657, 94.5107) knots 0 0 0 1 1 1
  line L1471 (-21.5257, 94.7506) -> (-21.5257, 94.5107) construction
  line L1472 (-21.5257, 94.5107) -> (-21.7657, 94.5107) construction
  line L1473 (-21.7657, 94.5107) -> (-22.4815, 94.5107)
  spline S399 degree 2 poles (-16.2592, 94.5107) (-16.6511, 94.5107) (-17.219, 95.0705) (-17.219, 95.4664) knots 0 0 0 1 2 2 2
  line L1474 (-16.2592, 94.5107) -> (-16.6511, 94.5107) construction
  line L1475 (-16.6511, 94.5107) -> (-17.219, 95.0705) construction
  line L1476 (-17.219, 95.0705) -> (-17.219, 95.4664) construction
  line L1477 (-17.219, 95.4664) -> (-17.219, 96.906)
  spline S400 degree 2 poles (-17.219, 96.906) (-17.219, 97.3019) (-16.6511, 97.8618) (-16.2592, 97.8618) knots 0 0 0 1 2 2 2
  line L1478 (-17.219, 96.906) -> (-17.219, 97.3019) construction
  line L1479 (-17.219, 97.3019) -> (-16.6511, 97.8618) construction
  line L1480 (-16.6511, 97.8618) -> (-16.2592, 97.8618) construction
  line L1481 (-16.2592, 97.8618) -> (-15.5434, 97.8618)
  spline S401 degree 2 poles (-15.5434, 97.8618) (-15.3035, 97.8618) (-15.3035, 97.6218) knots 0 0 0 1 1 1
  line L1482 (-15.5434, 97.8618) -> (-15.3035, 97.8618) construction
  line L1483 (-15.3035, 97.8618) -> (-15.3035, 97.6218) construction
  spline S402 degree 2 poles (-15.3035, 97.6218) (-15.3035, 97.3819) (-15.5434, 97.3819) knots 0 0 0 1 1 1
  line L1484 (-15.3035, 97.6218) -> (-15.3035, 97.3819) construction
  line L1485 (-15.3035, 97.3819) -> (-15.5434, 97.3819) construction
  line L1486 (-15.5434, 97.3819) -> (-16.2592, 97.3819)
  spline S403 degree 2 poles (-16.2592, 97.3819) (-16.4552, 97.3819) (-16.7391, 97.098) (-16.7391, 96.902) knots 0 0 0 1 2 2 2
  line L1487 (-16.2592, 97.3819) -> (-16.4552, 97.3819) construction
  line L1488 (-16.4552, 97.3819) -> (-16.7391, 97.098) construction
  line L1489 (-16.7391, 97.098) -> (-16.7391, 96.902) construction
  line L1490 (-16.7391, 96.902) -> (-16.7391, 95.4704)
  spline S404 degree 2 poles (-16.7391, 95.4704) (-16.7391, 95.2745) (-16.4552, 94.9906) (-16.2592, 94.9906) knots 0 0 0 1 2 2 2
  line L1491 (-16.7391, 95.4704) -> (-16.7391, 95.2745) construction
  line L1492 (-16.7391, 95.2745) -> (-16.4552, 94.9906) construction
  line L1493 (-16.4552, 94.9906) -> (-16.2592, 94.9906) construction
  line L1494 (-16.2592, 94.9906) -> (-15.5434, 94.9906)
  spline S405 degree 2 poles (-15.5434, 94.9906) (-15.3035, 94.9906) (-15.3035, 94.7506) knots 0 0 0 1 1 1
  line L1495 (-15.5434, 94.9906) -> (-15.3035, 94.9906) construction
  line L1496 (-15.3035, 94.9906) -> (-15.3035, 94.7506) construction
  spline S406 degree 2 poles (-15.3035, 94.7506) (-15.3035, 94.5107) (-15.5434, 94.5107) knots 0 0 0 1 1 1
  line L1497 (-15.3035, 94.7506) -> (-15.3035, 94.5107) construction
  line L1498 (-15.3035, 94.5107) -> (-15.5434, 94.5107) construction
  line L1499 (-15.5434, 94.5107) -> (-16.2592, 94.5107)
  spline S407 degree 2 poles (-8.1255, 96.906) (-8.1255, 97.102) (-8.4054, 97.3819) (-8.6014, 97.3819) knots 0 0 0 1 2 2 2
  line L1500 (-8.1255, 96.906) -> (-8.1255, 97.102) construction
  line L1501 (-8.1255, 97.102) -> (-8.4054, 97.3819) construction
  line L1502 (-8.4054, 97.3819) -> (-8.6014, 97.3819) construction
  line L1503 (-8.6014, 97.3819) -> (-9.0812, 97.3819)
  spline S408 degree 2 poles (-9.0812, 97.3819) (-9.2772, 97.3819) (-9.5571, 97.102) (-9.5571, 96.906) knots 0 0 0 1 2 2 2
  line L1504 (-9.0812, 97.3819) -> (-9.2772, 97.3819) construction
  line L1505 (-9.2772, 97.3819) -> (-9.5571, 97.102) construction
  line L1506 (-9.5571, 97.102) -> (-9.5571, 96.906) construction
  spline S409 degree 2 poles (-9.5571, 95.4704) (-9.5571, 95.2745) (-9.2732, 94.9906) (-9.0772, 94.9906) knots 0 0 0 1 2 2 2
  line L1507 (-9.5571, 95.4704) -> (-9.5571, 95.2745) construction
  line L1508 (-9.5571, 95.2745) -> (-9.2732, 94.9906) construction
  line L1509 (-9.2732, 94.9906) -> (-9.0772, 94.9906) construction
  line L1510 (-9.0772, 94.9906) -> (-7.8856, 94.9906)
  spline S410 degree 2 poles (-7.8856, 94.9906) (-7.6457, 94.9906) (-7.6457, 94.7506) knots 0 0 0 1 1 1
  line L1511 (-7.8856, 94.9906) -> (-7.6457, 94.9906) construction
  line L1512 (-7.6457, 94.9906) -> (-7.6457, 94.7506) construction
  spline S411 degree 2 poles (-7.6457, 94.7506) (-7.6457, 94.5107) (-7.8856, 94.5107) knots 0 0 0 1 1 1
  line L1513 (-7.6457, 94.7506) -> (-7.6457, 94.5107) construction
  line L1514 (-7.6457, 94.5107) -> (-7.8856, 94.5107) construction
  line L1515 (-7.8856, 94.5107) -> (-9.0812, 94.5107)
  spline S412 degree 2 poles (-9.0812, 94.5107) (-9.4771, 94.5107) (-10.037, 95.0705) (-10.037, 95.4664) knots 0 0 0 1 2 2 2
  line L1516 (-9.0812, 94.5107) -> (-9.4771, 94.5107) construction
  line L1517 (-9.4771, 94.5107) -> (-10.037, 95.0705) construction
  line L1518 (-10.037, 95.0705) -> (-10.037, 95.4664) construction
  line L1519 (-10.037, 95.4664) -> (-10.037, 96.906)
  spline S413 degree 2 poles (-10.037, 96.906) (-10.037, 97.3019) (-9.4771, 97.8618) (-9.0812, 97.8618) knots 0 0 0 1 2 2 2
  line L1520 (-10.037, 96.906) -> (-10.037, 97.3019) construction
  line L1521 (-10.037, 97.3019) -> (-9.4771, 97.8618) construction
  line L1522 (-9.4771, 97.8618) -> (-9.0812, 97.8618) construction
  line L1523 (-9.0812, 97.8618) -> (-8.6014, 97.8618)
  spline S414 degree 2 poles (-8.6014, 97.8618) (-8.2055, 97.8618) (-7.6457, 97.3019) (-7.6457, 96.906) knots 0 0 0 1 2 2 2
  line L1524 (-8.6014, 97.8618) -> (-8.2055, 97.8618) construction
  line L1525 (-8.2055, 97.8618) -> (-7.6457, 97.3019) construction
  line L1526 (-7.6457, 97.3019) -> (-7.6457, 96.906) construction
  line L1527 (-7.6457, 96.906) -> (-7.6457, 96.1862)
  spline S415 degree 2 poles (-7.6457, 96.1862) (-7.6457, 95.9463) (-7.8856, 95.9463) knots 0 0 0 1 1 1
  line L1528 (-7.6457, 96.1862) -> (-7.6457, 95.9463) construction